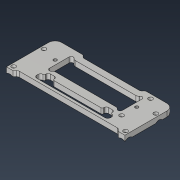
# Autodesk Inventor part: Dribbler Bruecke
Saved by Autodesk Inventor 2022.1 (Build 261234020, 234B)
## iProperties
Part Number: Dribbler Bruecke
Material: Aluminium 6061
Document SubType Name: Modeling
Designer: rYan
Mass: 19.5711 g
Surface Area: 60.4424 cm^2
Volume: 7.24854 cm^3
Density: 2.7 g/cm^3
Appearance: Aluminium - flach
Author: rYan
Autodesk Inventor part; units mm, degrees
ref_plane "YZ Plane" through (0, 0, 0) normal (1, 0, 0) x (0, 1, 0)
ref_plane "XZ Plane" through (0, 0, 0) normal (0, 1, 0) x (-1, 0, 0)
ref_plane "XY Plane" through (0, 0, 0) normal (0, 0, 1) x (1, 0, 0)
sketch "Skizze1" plane through (0, 0, 0) normal (0, 0, 1) x (1, 0, 0)
  line L0 (-45, 0) -> (45, 0)
  line L1 (45, 0) -> (45, -37)
  line L2 (-45, -37) -> (-45, 0)
  line L3 (40, -37) -> (40, -35)
  line L4 (-40, -35) -> (-40, -37)
  line L5 (45, -37) -> (40, -37)
  line L6 (-40, -37) -> (-45, -37)
  line L7 (0, 7.4) -> (0, -44.4) projected
  line L8 (-63, 0) -> (63, 0) projected
  line L9 (-42.5, -37) -> (-42.5, 0) construction
  line L10 (42.5, -37) -> (42.5, 0) construction
  line L11 (40, -35) -> (-40, -35)
  point P0 (0, 0)
  point P1 (-42.5, -11)
  point P2 (-42.5, -34)
  point P3 (42.5, -34)
  point P4 (42.5, -11)
  dimension "d0" = 90
  dimension "d1" = 37
  dimension "d3" = 5
  dimension "d24" = 2
  dimension "d39" = 23
  dimension "d40" = 3
  constraints: 20 end point, 6 point on line, 4 parallel, 3 perpendicular, 2 horizontal, 2 midpoint, 2 symmetric about line, 1 collinear, 3 other
  measures "d0" distance of L0.start L0.end
  measures "d1" distance of L2.start L0.start
  measures "d3" distance of L4.end L2.start
  measures "d24" distance of L3.start L3.end
  measures "d39" distance of point (-42.5, -34) point (-42.5, -11)
  measures "d40" distance from line of L6 point (-42.5, -34)
extrude "Extrusion1" add sketch "Skizze1" along normal blind 4
hole "Bohrung1" at (-42.5, -11, 0) at (-42.5, -34, 0) at (42.5, -34, 0) at (42.5, -11, 0) direction (0, 0, 1) diameter 3.2 end through all countersink diameter 7.2 countersink angle 90
sketch "Skizze3" plane through (0, 0, 4) normal (0, 0, 1) x (1, 0, 0)
  line L0 (0, 7.4) -> (0, -44.4) projected
  line L1 (-31, -14) -> (31, -14) construction
  line L2 (45, 0) -> (-45, 0) construction
  line L3 (-45, -37) -> (-40, -37) projected
  point P0 (0, 0)
  dimension "d15" = 62
  dimension "d42" = 23
  constraints: 2 coincident, 2 end point, 1 horizontal, 1 symmetric about line
  measures "d15" distance of L1.start L1.end
  measures "d42" distance between parallel lines of L1 L3
hole "Bohrung2" at (-31, -14, 4) at (31, -14, 4) direction (0, 0, -1) diameter 2.459 end through all thread size "M3x0.5" class "6H" standard "ISO Metric profile"
chamfer "Fase1" distance 2 angle 45 2 edges at (40, -35, 2.4537) (-40, -35, 2.4537)
sketch "Skizze4" plane through (0, 0, 0) normal (0, 0, -1) x (-1, 0, 0)
  line L0 (0, -44.4) -> (0, 7.4) projected
  line L1 (-35, -11.2401) -> (35, -11.2401) construction
  point P0 (0, 0)
  point P1 (0, -11.2401)
  dimension "d31" = 35
  constraints: 2 coincident, 2 end point, 1 horizontal, 1 midpoint, 1 point on line, 1 symmetric about line
  measures "d31" distance from line of L1.start L0
hole "Bohrung3" [suppressed]
sketch "Skizze5" plane through (0, 0, 0) normal (0, 0, -1) x (-1, 0, 0)
  line L0 (-40.51, -37) -> (-44.49, -37) projected
  line L1 (-45, -37) -> (-44.49, -37) projected
  line L2 (-40, -37) -> (-45, -37) projected
  line L3 (-40.51, -37) -> (-40, -37) projected
  line L4 (-30.7, -25.2) -> (-30.7, -3.2) construction
  line L5 (-45, -36.5904) -> (-45, -31.4096) projected
  line L6 (-45, -13.5904) -> (-45, -31.4096) projected
  line L7 (-45, -13.5904) -> (-45, -8.4096) projected
  line L8 (-45, 0) -> (-45, -8.4096) projected
  line L9 (-45, -37) -> (-45, 0) projected
  line L10 (-45, -36.5904) -> (-45, -37) projected
  point P0 (0, 0)
  point P1 (-30.7, -14.2)
  dimension "d44" = 22
  dimension "d45" = 14.3
  dimension "d65" = 22.8
  constraints: 2 coincident, 2 end point, 1 midpoint, 1 vertical
  measures "d44" distance of L4.start L4.end
  measures "d45" distance between parallel lines of L4 L9
  measures "d65" distance from line of point (-30.7, -14.2) L0
hole "Bohrung4" at (30.7, -25.2, 0) at (30.7, -3.2, 0) direction (0, 0, 1) diameter 3.2 end through all countersink diameter 7.2 countersink angle 90
sketch "Skizze6" plane through (0, 0, 0) normal (0, 0, -1) x (-1, 0, 0)
  line L0 (-36, -23.2) -> (-36, -5.2)
  line L1 (-40, -5.2) -> (-40, -23.2)
  line L2 (-24.5, -21.7) -> (24.5, -21.7)
  line L3 (27.7, -21.7) -> (27.7, -6.7)
  line L4 (24.5, -6.7) -> (-24.5, -6.7)
  line L5 (-27.7, -6.7) -> (-27.7, -21.7)
  circle A0 centre (-30.7, -25.2) radius 1.6 projected
  circle A1 centre (-30.7, -3.2) radius 1.6 projected
  circle A2 centre (-30.7, -25.2) radius 1.6 construction
  line L6 (-30.7, -25.2) -> (-30.7, -3.2) construction
  line L7 (0, -44.4) -> (0, 7.4) projected
  line L8 (-30.7, -14.2) -> (0, -14.2) construction
  arc A3 (-36, -5.2) -> (-40, -5.2) centre (-38, -5.2) ccw
  arc A4 (-40, -23.2) -> (-36, -23.2) centre (-38, -23.2) ccw
  line L9 (-45, 0) -> (-45, -8.4096) projected
  arc A5 (24.5, -21.7) -> (27.7, -21.7) centre (26.1, -21.7) ccw
  arc A6 (27.7, -6.7) -> (24.5, -6.7) centre (26.1, -6.7) ccw
  arc A7 (-27.7, -21.7) -> (-24.5, -21.7) centre (-26.1, -21.7) ccw
  arc A8 (-24.5, -6.7) -> (-27.7, -6.7) centre (-26.1, -6.7) ccw
  point P0 (0, 0)
  dimension "d63" = 3
  dimension "d66" = 15
  dimension "d68" = 4
  dimension "d69" = 18
  dimension "d70" = 5
  dimension "d73" = 1.6
  constraints: 16 end point, 12 point on circle, 8 tangent, 6 centre point, 3 parallel, 2 horizontal, 2 point on line, 1 midpoint, 1 perpendicular, 1 vertical, 6 other
  measures "d63" distance between parallel lines of L5 L6
  measures "d66" distance of L3.start L3.end
  measures "d68" distance between parallel lines of L1 L0
  measures "d69" distance of L0.start L0.end
  measures "d70" distance between parallel lines of L9 L1
  measures "d73" radius of A5
extrude "Extrusion2" cut sketch "Skizze6" against normal through all contours A7 L5 A8 L4 L7 L2 | L7 L4 A6 L3 A5 L2
fillet "Rundung3" radius 5 2 edges at (-45, 0, 2) (45, 0, 2)
fillet "Rundung4" radius 2 2 edges at (-38, -35, 2) (38, -35, 2)
fillet "Rundung5" radius 2 4 edges at (-24.5, -21.7, 2) (24.5, -21.7, 2) (24.5, -6.7, 2) (-24.5, -6.7, 2)
sketch "Skizze7" plane through (0, 0, 0) normal (0, 0, -1) x (-1, 0, 0)
  line L0 (40, 0) -> (-29.0508, 0) projected
  line L1 (0, -44.8) -> (0, 9.8) projected
  line L2 (21, 0) -> (-21, 0) construction
  line L3 (21, 2) -> (-21, 2)
  line L4 (-21, -2) -> (21, -2)
  arc A0 (21, -2) -> (21, 2) centre (21, 0) ccw
  arc A1 (-21, 2) -> (-21, -2) centre (-21, 0) ccw
  point P0 (0, 0)
  dimension "d75" = 4
  dimension "d76" = 42
  constraints: 8 end point, 4 point on circle, 4 tangent, 2 centre point, 1 midpoint, 1 parallel, 1 point on line
  measures "d75" diameter of A1
  measures "d76" distance of L4.start L4.end
extrude "Extrusion3" cut sketch "Skizze7" against normal through all
fillet "Rundung6" radius 2 2 edges at (-23, 0, 2) (23, 0, 2)
sketch "Skizze8" plane through (0, 0, 4) normal (0, 0, 1) x (1, 0, 0)
  line L0 (-26, -33) -> (26, -33)
  line L1 (0, 7.4) -> (0, -44.4) projected
  line L2 (-37.1716, -35) -> (37.1716, -35) projected
  line L3 (28, -31) -> (28, -30)
  line L4 (-28, -31) -> (-28, -30)
  line L5 (18.85, -28) -> (18.85, -26.6)
  line L6 (20.45, -25) -> (23.65, -25)
  line L7 (25.25, -26.6) -> (25.25, -28)
  line L8 (-18.85, -28) -> (-18.85, -26.6)
  line L9 (-20.45, -25) -> (-23.65, -25)
  line L10 (-25.25, -26.6) -> (-25.25, -28)
  line L11 (26, -28) -> (25.25, -28)
  line L12 (18.85, -28) -> (-18.85, -28)
  line L13 (-25.25, -28) -> (-26, -28)
  line L14 (22.05, -25) -> (22.05, -28.32) construction
  arc A0 (26, -33) -> (28, -31) centre (26, -31) ccw
  arc A1 (28, -30) -> (26, -28) centre (26, -30) ccw
  arc A2 (-28, -31) -> (-26, -33) centre (-26, -31) ccw
  arc A3 (-26, -28) -> (-28, -30) centre (-26, -30) ccw
  arc A4 (25.25, -26.6) -> (23.65, -25) centre (23.65, -26.6) ccw
  arc A5 (20.45, -25) -> (18.85, -26.6) centre (20.45, -26.6) ccw
  arc A6 (-18.85, -26.6) -> (-20.45, -25) centre (-20.45, -26.6) ccw
  arc A7 (-23.65, -25) -> (-25.25, -26.6) centre (-23.65, -26.6) ccw
  point P0 (0, 0)
  point P1 (28, -28)
  point P2 (-28, -28)
  point P3 (-28, -33)
  point P4 (28, -33)
  point P5 (18.85, -25)
  point P6 (25.25, -25)
  point P7 (-18.85, -25)
  point P8 (-25.25, -25)
  dimension "d80" = 2
  dimension "d85" = 22.05
  dimension "d86" = 6.4
  dimension "d87" = 56
  dimension "d88" = 5
  dimension "d89" = 3
  dimension "d90" = 2
  dimension "d91" = 1.6
  constraints: 26 end point, 17 point on line, 16 point on circle, 16 tangent, 8 centre point, 6 equal radius, 5 parallel, 4 vertical, 2 collinear, 1 midpoint, 4 other
  measures "d80" distance between parallel lines of L2 L0
  measures "d85" distance between parallel lines of L1 L14
  measures "d86" distance of point (18.85, -25) point (25.25, -25)
  measures "d87" distance of point (-28, -33) point (28, -33)
  measures "d88" distance between parallel lines of L0 L12
  measures "d89" distance of L5.start point (18.85, -25)
  measures "d90" radius of A0
  measures "d91" radius of A4
extrude "Extrusion4" cut sketch "Skizze8" against normal through all
fillet "Rundung7" radius 1 4 edges at (25.25, -28, 2) (18.85, -28, 2) (-18.85, -28, 2) (-25.25, -28, 2)
